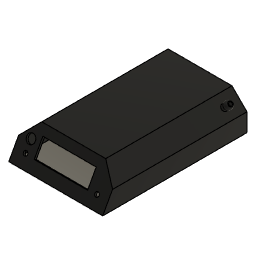
shutter-meter-fusion360 (Autodesk Fusion 360 design; units mm, degrees)
Autodesk Fusion 360 part; units mm, degrees
sketch "Sketch1" plane through (0, 0, 0) normal (0, 0, 1) x (1, 0, 0)
  line L0 (0, 0) -> (85, 0)
  line L1 (85, 0) -> (85, 160)
  line L2 (85, 160) -> (0, 160)
  line L3 (0, 160) -> (0, 0)
  dimension "d1" = 85
  dimension "d2" = 160
  constraint horizontal L0
  constraint vertical L1
  constraint horizontal L2
  constraint vertical L3
  constraint coincident L0.start L3.end
  measures "d1" distance of L0.start L0.end
  measures "d2" distance of L0.start L2.end
  measures "d6" distance of L0.start
  measures "d8" distance of L0.start
extrude "Extrude1" add sketch "Sketch1" along normal blind 44 contours L0 L1 L2 L3 picked at (28.333333, 106.666667) makes body 1
sketch "Sketch2" plane through (0, 0, 0) normal (0, 1, 0) x (1, 0, 0)
  line L0 (85.000001, -44.000001) -> (110.000001, -44.000001)
  line L1 (110.000001, -44.000001) -> (110.000001, 0)
  line L2 (110.000001, 0) -> (85.000001, 0)
  line L3 (85.000001, 0) -> (85.000001, -44.000001)
  line L4 (0, 0) -> (-25, 0)
  line L5 (-25, 0) -> (-25, -44)
  line L6 (-25, -44) -> (0, -44)
  line L7 (0, -44) -> (0, 0)
  dimension "d5" = 25
  dimension "d6" = 44.000001
  dimension "d7" = 25
  dimension "d8" = 44
  constraint horizontal L0
  constraint vertical L1
  constraint horizontal L2
  constraint vertical L3
  constraint horizontal L4
  constraint vertical L5
  constraint horizontal L6
  constraint vertical L7
  constraint coincident L4.start L7.end
  measures "d7" distance of L4.start L4.end
  measures "d8" distance of L4.start L6.end
extrude "Extrude2" add sketch "Sketch2" along normal blind 160 contours L0 L1 L2 L3 picked at (93.333335, -14.666667) bodies 1
extrude "Extrude3" add sketch "Sketch2" along normal blind 160 contours L4 L5 L6 L7 picked at (-16.666667, -14.666667) bodies 1
move_face "OffsetFaces1" offset -5 1 faces at (110.000001, 53.333333, 29.333334) on bodies 1
move_face "OffsetFaces2" offset -5 1 faces at (-25, 106.666667, 29.333333) on bodies 1
chamfer "Chamfer1" distance 20 angle 45 2 edges at (105.000001, 80, 44) (-20, 80, 44) on bodies 1
move_face "OffsetFaces3" offset 32 1 faces at (28.333334, 0, 14.666667) on bodies 1
chamfer "Chamfer2" distance 24 distance2 44 1 edges at (42.500001, -32, 44) measured on face at (28.333333, 42.666667, 44) on bodies 1
sketch "Sketch3" plane through (0, -24.66242, 13.452229) normal (0, -0.877896, 0.478852) x (1, 0, 0)
  line L0 (105.000001, 12.014835) -> (85.000001, 34.796588)
  line L1 (85.000001, 34.796588) -> (0, 34.796588)
  line L2 (0, 34.796588) -> (-20, 12.014835)
  line L3 (-20, 12.014835) -> (-20, -15.323268)
  line L4 (-20, -15.323268) -> (105.000001, -15.323268)
  line L5 (105.000001, -15.323268) -> (105.000001, 12.014835)
  line L6 (42.500001, 34.796588) -> (42.500001, 24.796588)
  line L7 (42.500001, 24.796588) -> (6.930001, 24.796588)
  line L8 (42.500001, 24.796588) -> (78.070001, 24.796588)
  line L9 (6.930001, 24.796588) -> (78.070001, 24.796588)
  line L10 (78.070001, 24.796588) -> (78.070001, 0.696588)
  line L11 (78.070001, 0.696588) -> (6.930001, 0.696588)
  line L12 (6.930001, 0.696588) -> (6.930001, 24.796588)
  dimension "d19" = 10
  dimension "d22" = 35.57
  dimension "d23" = 35.57
  dimension "d24" = 71.14
  dimension "d25" = 24.1
  constraint perpendicular L1 L6
  constraint perpendicular L6 L7
  constraint perpendicular L6 L8
  constraint horizontal L9
  constraint vertical L10
  constraint horizontal L11
  constraint vertical L12
shell "Shell1" thickness 3 removed faces 2 at (56.666667, 96, 0) at (95.000001, -32, 0) on bodies 1
extrude "Extrude4" cut sketch "Sketch3" against normal blind 10 contours L7 L8 L9 L10 L11 L12 picked at (42.500001, 8.729921) bodies 1
copy_body "Body->Comp1" bodies 1 removing the originals makes body 2 in component "Case"
sketch "Sketch1 (2)" plane through (0, -24.66242, 13.452229) normal (0, -0.877896, 0.478852) x (1, 0, 0) in component "Case"
  line L0 (105.000001, 12.014835) -> (85.000001, 34.796588)
  line L1 (85.000001, 34.796588) -> (0, 34.796588)
  line L2 (0, 34.796588) -> (-20, 12.014835)
  line L3 (-20, 12.014835) -> (-20, -15.323268)
  line L4 (-20, -15.323268) -> (105.000001, -15.323268)
  line L5 (105.000001, -15.323268) -> (105.000001, 12.014835)
  line L6 (6, 25) -> (80.000001, 25)
  line L7 (80.000001, 25) -> (80.000001, 0)
  line L8 (80.000001, 0) -> (6, 0)
  line L9 (6, 0) -> (6, 25)
  point P0 (78.070001, 24.796588)
  constraint horizontal L6
  constraint vertical L7
  constraint horizontal L8
  constraint vertical L9
extrude "Extrude1'" add sketch "Sketch1 (2)" against normal blind 3 contours L6 L7 L8 L9 picked at (30.666667, 16.666667) bodies 2 in component "Case"
sketch "Ball Joint" plane through (0, 0, 0) normal (0, 1, 0) x (1, 0, 0) in component "Arm base"
  line L0 (0, 0) -> (0, -13)
  line L1 (0, 0) -> (4.05, 0)
  line L2 (0, -13) -> (0, -14)
  circle A0 centre (0, -8.9) radius 5.1
  line L3 (4.05, 0) -> (4.05, -5.800403)
  line L4 (0, -13) -> (3.03315, -13)
  line L5 (0, -13) -> (2, -13)
  line L6 (2, -13) -> (2, 0)
  line L7 (2, 0) -> (0, 0)
  line L8 (0, 0) -> (0, -13)
  dimension "d29" = 13
  dimension "d31" = 4.05
  dimension "d32" = 1
  dimension "d33" = 10.2
  dimension "d34" = 2
  constraint coincident L0.start L1.start
  constraint vertical L0
  constraint perpendicular L0 L1
  constraint parallel L0 L2
  constraint coincident L2.end A0
  constraint perpendicular L1 L3
  constraint perpendicular L2 L4
  constraint horizontal L5
  constraint vertical L6
  constraint horizontal L7
  constraint vertical L8
  measures "d29" distance of L0.start L0.end
  measures "d31" distance of L0.start L1.end
  measures "d32" distance of L0.end L2.end
  measures "d33" diameter of A0
  measures "d34" distance of L0.end L5.end
revolve "Revolve1" add sketch "Ball Joint" angle 360 about axis through (0, 0, 0) along (0, 0, 1) separate body contours L1 A0 L3 L6 | A0 L4 L6 picked at (2.683333, -1.402839) picked at (2.195115, -7.237462) makes body 3 in component "Arm base"
move_body "Move1" bodies 3 to x (0.70710678, 0, -0.70710678) y (0, 1, 0) z (0.70710678, 0, 0.70710678) at (0, 0, 0) in component "Arm base"
move_body "Move2" bodies 3 to x (1, 0, 0) y (0, 1, 0) z (0, 0, 1) at (96.414215, 160, 35.414214) in component "Arm base"
move_body "Move3" bodies 3 to x (1, 0, 0) y (0, 1, 0) z (0, 0, 1) at (-1.414214, 0, -1.414214) in component "Arm base"
move_body "Move4" bodies 3 to x (1, 0, 0) y (0, 1, 0) z (0, 0, 1) at (0, -28, 0) in component "Arm base"
sketch "Sketch1 (1)" plane through (64.500001, 0, 64.500001) normal (0.707107, 0, 0.707107) x (0, 1, 0) in component "Case"
  line L0 (-8, -28.991379) -> (-18.909091, -57.27565)
  line L1 (-18.909091, -57.27565) -> (160, -57.27565)
  line L2 (160, -57.27565) -> (160, -28.991378)
  line L3 (160, -28.991378) -> (-8, -28.991379)
  line L4 (160, -43.133514) -> (140, -43.133514)
  dimension "d40" = 20
  constraint perpendicular L2 L4
hole "Hole1" at (95.000001, 140, 34) direction (-0.707107, 0, -0.707107) diameter 4 depth 3 tip angle 180 counterbore diameter 8.12 counterbore depth 1.5 bodies 2 in component "Case"
sketch "Sketch2 (2)" plane through (-22, 0, 22) normal (-0.707107, 0, 0.707107) x (0, -1, 0) in component "Case"
  line L0 (18.909091, 2.828427) -> (8, 31.112698)
  line L1 (8, 31.112698) -> (-160, 31.112699)
  line L2 (-160, 31.112699) -> (-160, 2.828427)
  line L3 (-160, 2.828427) -> (18.909091, 2.828427)
  line L4 (-160, 16.970563) -> (-140, 16.970563)
  dimension "d46" = 20
  constraint perpendicular L2 L4
hole "Hole2" at (-10, 140, 34) direction (0.707107, 0, -0.707107) diameter 4 depth 3 tip angle 180 counterbore diameter 8.12 counterbore depth 1.5 bodies 2 in component "Case"
move_body "Move5" bodies 3 to x (1, 0, 0) y (0, 1, 0) z (0, 0, 1) at (0, 8, 0) in component "Arm base"
move_body "Move6" bodies 3 to x (1, 0, 0) y (0, 1, 0) z (0, 0, 1) at (-1.06066, 0, -1.06066) in component "Arm base"
sketch "Sketch3 (2)" plane through (0, -22.028734, 12.015673) normal (0, 0.877896, -0.478852) x (-1, 0, 0) in component "Case"
  line L0 (-83.757361, 33.015689) -> (-102.000001, 12.235722)
  line L1 (-102.000001, 12.235722) -> (-102.000001, -13.686905)
  line L2 (-102.000001, -13.686905) -> (17, -13.686905)
  line L3 (17, -13.686905) -> (17, 12.235722)
  line L4 (17, 12.235722) -> (-1.242641, 33.015689)
  line L5 (-1.242641, 33.015689) -> (-83.757361, 33.015689)
  line L6 (-78.000001, 23.015689) -> (-7.000001, 23.015689)
  line L7 (-7.000001, 23.015689) -> (-7.000001, -0.984311)
  line L8 (-7.000001, -0.984311) -> (-78.000001, -0.984311)
  line L9 (-78.000001, -0.984311) -> (-78.000001, 23.015689)
  line L10 (-82.500001, 23.015689) -> (-82.500001, 29.515689)
  line L11 (-82.500001, 29.515689) -> (-78.000001, 29.515689)
  line L12 (-82.500001, 29.515689) -> (-2.500001, 29.515689)
  line L13 (-2.500001, 29.515689) -> (-2.500001, -6.484311)
  line L14 (-2.500001, -6.484311) -> (-82.500001, -6.484311)
  line L15 (-82.500001, -6.484311) -> (-82.500001, 29.515689)
  line L16 (-82.500001, 29.515689) -> (-80.400001, 29.515689)
  line L17 (-80.400001, 29.515689) -> (-80.400001, 27.415689)
  line L18 (-80.400001, 27.415689) -> (-82.500001, 27.415689)
  line L19 (-82.500001, 27.415689) -> (-82.500001, 29.515689)
  line L20 (-82.500001, -6.484311) -> (-80.400001, -6.484311)
  line L21 (-80.400001, -6.484311) -> (-80.400001, -4.384311)
  line L22 (-80.400001, -4.384311) -> (-82.500001, -4.384311)
  line L23 (-82.500001, -4.384311) -> (-82.500001, -6.484311)
  line L24 (-2.500001, -6.484311) -> (-4.600001, -6.484311)
  line L25 (-4.600001, -6.484311) -> (-4.600001, -4.384311)
  line L26 (-4.600001, -4.384311) -> (-2.500001, -4.384311)
  line L27 (-2.500001, -4.384311) -> (-2.500001, -6.484311)
  line L28 (-2.500001, 29.515689) -> (-4.600001, 29.515689)
  line L29 (-4.600001, 29.515689) -> (-4.600001, 27.415689)
  line L30 (-4.600001, 27.415689) -> (-2.500001, 27.415689)
  line L31 (-2.500001, 27.415689) -> (-2.500001, 29.515689)
  circle A0 centre (-80.400001, 27.415689) radius 2.05
  circle A1 centre (-80.400001, -4.384311) radius 2.05
  circle A2 centre (-4.600001, -4.384311) radius 2.05
  circle A3 centre (-4.600001, 27.415689) radius 2.05
  circle A4 centre (4.999999, 15.015689) radius 5.825
  circle A5 centre (-90.000001, 0.015689) radius 2.825
  circle A6 centre (5, 0.015689) radius 2.825
  dimension "d74" = 71
  dimension "d75" = 24
  dimension "d76" = 4.5
  dimension "d77" = 6.5
  dimension "d78" = 80
  dimension "d79" = 36
  dimension "d80" = 2.1
  dimension "d81" = 2.1
  dimension "d82" = 2.1
  dimension "d83" = 2.1
  dimension "d84" = 2.1
  dimension "d85" = 2.1
  dimension "d86" = 2.1
  dimension "d87" = 2.1
  dimension "d88" = 4.1
  dimension "d89" = 4.1
  dimension "d90" = 4.1
  dimension "d91" = 4.1
  dimension "d94" = 11.65
  dimension "d95" = 5.65
  dimension "d96" = 5.65
  constraint horizontal L6
  constraint vertical L7
  constraint horizontal L8
  constraint vertical L9
  constraint vertical L10
  constraint horizontal L11
  constraint horizontal L12
  constraint vertical L13
  constraint horizontal L14
  constraint vertical L15
  constraint horizontal L16
  constraint vertical L17
  constraint horizontal L18
  constraint vertical L19
  constraint horizontal L20
  constraint vertical L21
  constraint horizontal L22
  constraint vertical L23
  constraint horizontal L24
  constraint vertical L25
  constraint horizontal L26
  constraint vertical L27
  constraint horizontal L28
  constraint vertical L29
  constraint horizontal L30
  constraint vertical L31
  measures "d88" diameter of A0
  measures "d89" diameter of A1
  measures "d90" diameter of A2
  measures "d91" diameter of A3
  measures "d94" diameter of A4
  measures "d95" diameter of A5
  measures "d96" diameter of A6
extrude "Extrude2'" cut sketch "Sketch3 (2)" against normal blind 3 contours L6 L7 L8 L9 picked at (-54.333334, 15.015689) bodies 2 in component "Case"
extrude "Extrude3'" add sketch "Sketch3 (2)" along normal blind 6 contours L17 L18 A0 | L17 L18 A0 | L21 L22 A1 | L21 L22 A1 | L25 L26 A2 | L25 L26 A2 | L29 L30 A3 | L29 L30 A3 picked at (-81.759712, 27.512937) picked at (-80.400001, 26.052844) picked at (-80.400001, -3.021466) picked at (-81.759712, -4.48156) picked at (-5.490251, -3.352263) picked at (-3.240289, -4.48156) picked at (-3.267969, 27.705455) picked at (-3.328365, 26.925165) bodies 2 in component "Case"
hole "Hole3" at (80.400001, -3.633299, 33.210672) direction (0, -0.877896, 0.478852) diameter 2 depth 6 tip angle 180 bodies 2 in component "Case"
hole "Hole4" at (80.400001, -18.860797, 5.293593) direction (0, -0.877896, 0.478852) diameter 2 depth 6 tip angle 180 bodies 2 in component "Case"
hole "Hole5" at (4.600001, -18.860797, 5.293593) direction (0, -0.877896, 0.478852) diameter 2 depth 6 tip angle 180 bodies 2 in component "Case"
hole "Hole6" at (4.600001, -3.633299, 33.210672) direction (0, -0.877896, 0.478852) diameter 2 depth 6 tip angle 180 bodies 2 in component "Case"
sketch "Sketch4" plane through (0, 0, 0) normal (0, 0, -1) x (1, 0, 0) in component "Case"
  line L0 (-17, 28.582737) -> (102.000001, 28.582737)
  line L1 (102.000001, 28.582737) -> (102.000001, -157)
  line L2 (102.000001, -157) -> (-17, -157)
  line L3 (-17, -157) -> (-17, 28.582737)
  line L4 (-20, -160) -> (105.000001, -160)
  line L5 (105.000001, -160) -> (105.000001, 32)
  line L6 (105.000001, 32) -> (-20, 32)
  line L7 (-20, 32) -> (-20, -160)
  line L8 (-17, 28.582737) -> (-11, 28.582737)
  line L9 (-11, 28.582737) -> (-11, 22.582737)
  line L10 (-11, 22.582737) -> (-17, 22.582737)
  line L11 (-17, 22.582737) -> (-17, 28.582737)
  line L12 (-17, -157) -> (-11, -157)
  line L13 (-11, -157) -> (-11, -151)
  line L14 (-11, -151) -> (-17, -151)
  line L15 (-17, -151) -> (-17, -157)
  line L16 (102.000001, -157) -> (96.000001, -157)
  line L17 (96.000001, -157) -> (96.000001, -151)
  line L18 (96.000001, -151) -> (102.000001, -151)
  line L19 (102.000001, -151) -> (102.000001, -157)
  line L20 (102.000001, 28.563611) -> (96.000001, 28.563611)
  line L21 (96.000001, 28.563611) -> (96.000001, 22.563611)
  line L22 (96.000001, 22.563611) -> (102.000001, 22.563611)
  line L23 (102.000001, 22.563611) -> (102.000001, 28.563611)
  line L24 (-17, -64.208631) -> (-11, -64.208631)
  line L25 (-11, -64.208631) -> (-11, -61.208631)
  line L26 (-11, -61.208631) -> (-17, -61.208631)
  line L27 (-17, -61.208631) -> (-17, -64.208631)
  line L28 (-17, -64.208631) -> (-11, -64.208631)
  line L29 (-11, -64.208631) -> (-11, -67.208631)
  line L30 (-11, -67.208631) -> (-17, -67.208631)
  line L31 (-17, -67.208631) -> (-17, -64.208631)
  line L32 (102.000001, -64.208631) -> (96.000001, -64.208631)
  line L33 (96.000001, -64.208631) -> (96.000001, -61.208631)
  line L34 (96.000001, -61.208631) -> (102.000001, -61.208631)
  line L35 (102.000001, -61.208631) -> (102.000001, -64.208631)
  line L36 (102.000001, -64.208631) -> (96.000001, -64.208631)
  line L37 (96.000001, -64.208631) -> (96.000001, -67.208631)
  line L38 (96.000001, -67.208631) -> (102.000001, -67.208631)
  line L39 (102.000001, -67.208631) -> (102.000001, -64.208631)
  line L40 (-17, 28.582737) -> (102.000001, 28.582737)
  line L41 (102.000001, 28.582737) -> (102.000001, -157)
  line L42 (102.000001, -157) -> (-17, -157)
  line L43 (-17, -157) -> (-17, 28.582737)
  line L44 (103.500001, 30.082737) -> (103.500001, -158.5)
  line L45 (103.500001, -158.5) -> (-18.5, -158.5)
  line L46 (-18.5, -158.5) -> (-18.5, 30.082737)
  line L47 (-18.5, 30.082737) -> (103.500001, 30.082737)
  dimension "d113" = 6
  dimension "d114" = 6
  dimension "d115" = 6
  dimension "d116" = 6
  dimension "d117" = 6
  dimension "d118" = 6
  dimension "d119" = 6
  dimension "d120" = 6
  dimension "d121" = 6
  dimension "d122" = 3
  dimension "d123" = 6
  dimension "d124" = 3
  dimension "d125" = 6
  dimension "d126" = 3
  dimension "d127" = 6
  dimension "d128" = 3
  dimension "d131" = -1.5
  constraint horizontal L8
  constraint vertical L9
  constraint horizontal L10
  constraint vertical L11
  constraint horizontal L12
  constraint vertical L13
  constraint horizontal L14
  constraint vertical L15
  constraint coincident L2.end L3.start
  constraint horizontal L16
  constraint vertical L17
  constraint horizontal L18
  constraint vertical L19
  constraint horizontal L20
  constraint vertical L21
  constraint horizontal L22
  constraint vertical L23
  constraint horizontal L24
  constraint vertical L25
  constraint horizontal L26
  constraint vertical L27
  constraint horizontal L28
  constraint vertical L29
  constraint horizontal L30
  constraint vertical L31
  constraint horizontal L32
  constraint vertical L33
  constraint horizontal L34
  constraint vertical L35
  constraint horizontal L36
  constraint vertical L37
  constraint horizontal L38
  constraint vertical L39
  constraint horizontal L40
  constraint vertical L41
  constraint horizontal L42
  constraint vertical L43
  measures "d115" distance of L2.end L12.end
  measures "d116" distance of L2.end L14.end
extrude "Extrude4'" add sketch "Sketch4" against normal blind 10 contours L0 L3 L8 L9 L10 L11 L40 L43 | L3 L24 L25 L26 L27 L28 L43 | L1 L20 L21 L22 L23 L41 | L3 L24 L28 L29 L30 L31 L43 | L1 L32 L33 L34 L35 L36 L41 | L2 L3 L12 L13 L14 L15 L42 L43 | L1 L32 L36 L37 L38 L39 L41 | L1 L2 L16 L17 L18 L19 L41 L42 picked at (-15, 24.582737) picked at (-13, -62.208631) picked at (98.000001, 24.563611) picked at (-15, -66.208631) picked at (100.000001, -63.208631) picked at (-15, -153) picked at (98.000001, -66.208631) picked at (98.000001, -153) bodies 2 in component "Case"
extrude "Extrude5" cut sketch "Sketch4" against normal blind 1.5 contours L0 L3 L8 L9 L10 L11 L40 L43 | L0 L1 L2 L3 L9 L10 L13 L14 L17 L18 L20 L21 L22 L25 L26 L29 L30 L33 L34 L37 L38 L40 L41 L42 L43 | L3 L24 L25 L26 L27 L28 L43 | L1 L20 L21 L22 L23 L41 | L3 L24 L28 L29 L30 L31 L43 | L1 L32 L33 L34 L35 L36 L41 | L2 L3 L12 L13 L14 L15 L42 L43 | L1 L32 L36 L37 L38 L39 L41 | L1 L2 L16 L17 L18 L19 L41 L42 | L44 L45 L46 L47 picked at (-15, 24.582737) picked at (24.666667, -5.354094) picked at (-13, -62.208631) picked at (98.000001, 24.563611) picked at (-15, -66.208631) picked at (100.000001, -63.208631) picked at (-15, -153) picked at (98.000001, -66.208631) picked at (98.000001, -153) picked at (103.000001, -64.208631) bodies 2 in component "Case"
chamfer "Chamfer1'" distance 6 angle 45 1 edges at (102.000001, 64.208631, 10) on bodies 2 in component "Case"
chamfer "Chamfer2'" distance 6 angle 45 1 edges at (-17, 64.208631, 10) on bodies 2 in component "Case"
chamfer "Chamfer3" distance 6 angle 45 1 edges at (-17, 154, 10) on bodies 2 in component "Case"
chamfer "Chamfer4" distance 6 angle 45 1 edges at (102.000001, 154, 10) on bodies 2 in component "Case"
delete_face "DeleteFace1" 2 faces at (-13, -28.582737, 7.509988) (-17, -27.903643, 8.754994) on bodies 2 in component "Case"
delete_face "DeleteFace2" 1 faces at (100.000001, -28.563611, 7.533365) on bodies 2 in component "Case"
sketch "Sketch5" plane through (0, 0, 1.5) normal (0, 0, -1) x (1, 0, 0) in component "Case"
  line L0 (96.000001, -151) -> (96.000001, -157)
  line L1 (96.000001, -157) -> (-11, -157)
  line L2 (-11, -157) -> (-11, -151)
  line L3 (-11, -151) -> (-17, -151)
  line L4 (-17, -151) -> (-17, -67.208631)
  line L5 (-17, -67.208631) -> (-11, -67.208631)
  line L6 (-11, -67.208631) -> (-11, -61.208631)
  line L7 (-11, -61.208631) -> (-17, -61.208631)
  line L8 (-17, -61.208631) -> (-17, 22.582737)
  line L9 (-17, 22.582737) -> (-11, 22.582737)
  line L10 (-11, 22.582737) -> (-11, 27.764555)
  line L11 (-11, 27.764555) -> (96.000001, 27.764555)
  line L12 (96.000001, 27.764555) -> (96.000001, 22.563611)
  line L13 (96.000001, 22.563611) -> (102.000001, 22.563611)
  line L14 (102.000001, 22.563611) -> (102.000001, -61.208631)
  line L15 (102.000001, -61.208631) -> (96.000001, -61.208631)
  line L16 (96.000001, -61.208631) -> (96.000001, -67.208631)
  line L17 (96.000001, -67.208631) -> (102.000001, -67.208631)
  line L18 (102.000001, -67.208631) -> (102.000001, -151)
  line L19 (102.000001, -151) -> (96.000001, -151)
  line L20 (-18.5, 30.082737) -> (-18.5, -158.5)
  line L21 (-18.5, -158.5) -> (103.500001, -158.5)
  line L22 (103.500001, -158.5) -> (103.500001, 30.082737)
  line L23 (103.500001, 30.082737) -> (-18.5, 30.082737)
  line L24 (-11, -151) -> (-14, -151)
  line L25 (-14, -151) -> (-14, -154)
  line L26 (-14, -154) -> (-11, -154)
  line L27 (-11, -154) -> (-11, -151)
  line L28 (96.000001, -151) -> (99.000001, -151)
  line L29 (99.000001, -151) -> (99.000001, -154)
  line L30 (99.000001, -154) -> (96.000001, -154)
  line L31 (96.000001, -154) -> (96.000001, -151)
  line L32 (-11, -64.208631) -> (-14, -64.208631)
  line L33 (96.000001, -64.208631) -> (99.000001, -64.208631)
  line L34 (-11, 22.582737) -> (-14, 22.582737)
  line L35 (-14, 22.582737) -> (-14, 25.582737)
  line L36 (-14, 25.582737) -> (-11, 25.582737)
  line L37 (-11, 25.582737) -> (-11, 22.582737)
  line L38 (96.000001, 22.563611) -> (99.000001, 22.563611)
  line L39 (99.000001, 22.563611) -> (99.000001, 25.563611)
  line L40 (99.000001, 25.563611) -> (96.000001, 25.563611)
  line L41 (96.000001, 25.563611) -> (96.000001, 22.563611)
  dimension "d139" = 3
  dimension "d140" = 3
  dimension "d141" = 3
  dimension "d142" = 3
  dimension "d143" = 3
  dimension "d144" = 3
  dimension "d145" = 3
  dimension "d146" = 3
  dimension "d147" = 3
  dimension "d148" = 3
  constraint horizontal L24
  constraint vertical L25
  constraint horizontal L26
  constraint vertical L27
  constraint coincident L2.end L3.start
  constraint horizontal L28
  constraint vertical L29
  constraint horizontal L30
  constraint vertical L31
  constraint perpendicular L6 L32
  constraint perpendicular L16 L33
  constraint horizontal L34
  constraint vertical L35
  constraint horizontal L36
  constraint vertical L37
  constraint horizontal L38
  constraint vertical L39
  constraint horizontal L40
  constraint vertical L41
  measures "d139" distance of L2.end L24.end
  measures "d140" distance of L2.end L26.end
hole "Hole7" at (-14, -25.582737, 1.5) at (99.000001, -25.563611, 1.5) at (99.000001, 64.208631, 1.5) at (-14, 64.208631, 1.5) at (-14, 154, 1.5) at (99.000001, 154, 1.5) direction (0, 0, 1) diameter 2 depth 6 tip angle 180 bodies 2 in component "Case"
extrude "Extrude6" cut sketch "Sketch3 (2)" against normal blind 3 contours A4 | A5 | A6 picked at (6.539703, 15.247762) picked at (-90.765677, -0.124659) picked at (4.120269, 0.025024) bodies 2 in component "Case"
sketch "Sketch4 (2)" plane through (0, 0, 1.5) normal (0, 0, -1) x (1, 0, 0)
  circle A0 centre (-14, -154) radius 1
  circle A1 centre (99.000001, -64.208631) radius 1
  circle A2 centre (-14, 25.582737) radius 1
  circle A3 centre (99.000001, 25.563611) radius 1
  circle A4 centre (-14, -64.208631) radius 1
  circle A5 centre (99.000001, -154) radius 1
  line L0 (96.000001, -151) -> (96.000001, -157)
  line L1 (96.000001, -157) -> (-11, -157)
  line L2 (-11, -157) -> (-11, -151)
  line L3 (-11, -151) -> (-17, -151)
  line L4 (-17, -151) -> (-17, -67.208631)
  line L5 (-17, -67.208631) -> (-11, -67.208631)
  line L6 (-11, -67.208631) -> (-11, -61.208631)
  line L7 (-11, -61.208631) -> (-17, -61.208631)
  line L8 (-17, -61.208631) -> (-17, 22.582737)
  line L9 (-17, 22.582737) -> (-11, 22.582737)
  line L10 (-11, 22.582737) -> (-11, 27.764555)
  line L11 (-11, 27.764555) -> (96.000001, 27.764555)
  line L12 (96.000001, 27.764555) -> (96.000001, 22.563611)
  line L13 (96.000001, 22.563611) -> (102.000001, 22.563611)
  line L14 (102.000001, 22.563611) -> (102.000001, -61.208631)
  line L15 (102.000001, -61.208631) -> (96.000001, -61.208631)
  line L16 (96.000001, -61.208631) -> (96.000001, -67.208631)
  line L17 (96.000001, -67.208631) -> (102.000001, -67.208631)
  line L18 (102.000001, -67.208631) -> (102.000001, -151)
  line L19 (102.000001, -151) -> (96.000001, -151)
  line L20 (-18.5, 30.082737) -> (-18.5, -158.5)
  line L21 (-18.5, -158.5) -> (103.500001, -158.5)
  line L22 (103.500001, -158.5) -> (103.500001, 30.082737)
  line L23 (103.500001, 30.082737) -> (-18.5, 30.082737)
  line L24 (-18.5, 30.082737) -> (103.500001, 30.082737)
  line L25 (103.500001, 30.082737) -> (103.500001, -158.5)
  line L26 (103.500001, -158.5) -> (-18.5, -158.5)
  line L27 (-18.5, -158.5) -> (-18.5, 30.082737)
  constraint horizontal L24
  constraint vertical L25
  constraint horizontal L26
  constraint vertical L27
extrude "Extrude5'" add sketch "Sketch4 (2)" along normal blind 1.5 separate body contours L0 L1 L2 L3 L4 L5 L6 L7 L8 L9 L10 L11 L12 L13 L14 L15 L16 L17 L18 L19 | L20 L21 L22 L23 L24 L25 L26 L27 picked at (24.666667, -5.354094) picked at (99.574175, -156.824976) makes body 4
copy_body "Body->Comp2" bodies 4 removing the originals makes body 5 in component "BasePlate"
hole "Hole1'" at (99.000001, -25.563611, 0) direction (0, 0, 1) diameter 2 depth 4 tip angle 118 counterbore diameter 3.65 counterbore depth 1 bodies 5 in component "BasePlate"
hole "Hole2'" at (99.000001, 64.208631, 0) direction (0, 0, 1) diameter 2 depth 4 tip angle 118 counterbore diameter 3.65 counterbore depth 1 bodies 5 in component "BasePlate"
hole "Hole3'" at (99.000001, 154, 0) direction (0, 0, 1) diameter 2 depth 4 tip angle 118 counterbore diameter 3.65 counterbore depth 1 bodies 5 in component "BasePlate"
hole "Hole4'" at (-14, 154, 0) direction (0, 0, 1) diameter 2 depth 4 tip angle 118 counterbore diameter 3.65 counterbore depth 1 bodies 5 in component "BasePlate"
hole "Hole5'" at (-14, 64.208631, 0) direction (0, 0, 1) diameter 2 depth 4 tip angle 118 counterbore diameter 3.65 counterbore depth 1 bodies 5 in component "BasePlate"
hole "Hole6'" at (-14, -25.582737, 0) direction (0, 0, 1) diameter 2 depth 4 tip angle 118 counterbore diameter 3.65 counterbore depth 1 bodies 5 in component "BasePlate"
component "Arm base" placed x (1, 0, 0) y (0, 1, 0) z (0, 0, 1) at (0, 0, 0)
component "Case" placed x (1, 0, 0) y (0, 1, 0) z (0, 0, 1) at (0, 0, 0)
component "BasePlate" placed x (1, 0, 0) y (0, 1, 0) z (0, 0, 1) at (0, 0, 0)
